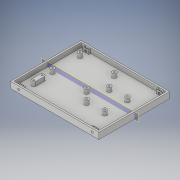
# Autodesk Inventor part: base
Saved by Autodesk Inventor 2017 (Build 210142000, 142)
## iProperties
Created: 2018-02-14
Part Number: base
Material: Generic
Document SubType Name: Modeling
Designer: chuck
Density: 1 g/cm^3
Appearance: Default
Author: chuck
Autodesk Inventor part; units mm, degrees
ref_plane "YZ Plane" through (0, 0, 0) normal (1, 0, 0) x (0, 1, 0)
ref_plane "XZ Plane" through (0, 0, 0) normal (0, 1, 0) x (-1, 0, 0)
ref_plane "XY Plane" through (0, 0, 0) normal (0, 0, 1) x (1, 0, 0)
sketch "Sketch1" plane through (0, 0, 0) normal (0, 1, 0) x (-1, 0, 0)
  line L0 (52.048, 52.048) -> (-82.4958, 52.048)
  line L1 (-82.4958, 52.048) -> (-82.4958, -55.394)
  line L2 (-82.4958, -55.394) -> (52.048, -55.394)
  line L3 (52.048, -55.394) -> (52.048, 52.048)
  line L4 (49.508, 49.508) -> (-79.9558, 49.508)
  line L5 (-79.9558, 49.508) -> (-79.9558, -52.854)
  line L6 (-79.9558, -52.854) -> (49.508, -52.854)
  line L7 (49.508, -52.854) -> (49.508, 49.508)
  point P0 (0, 0)
  dimension "d0" = 107.442
  dimension "d1" = 134.5438
  dimension "d2" = 2.54
  dimension "d3" = 2.54
  dimension "d4" = 2.54
  dimension "d5" = 2.54
  constraints: 16 end point, 4 parallel, 2 horizontal, 2 perpendicular
  measures "d0" distance of L2.end L0.start
  measures "d1" distance of L0.start L0.end
  measures "d2" distance between parallel lines of L2 L6
  measures "d3" distance between parallel lines of L3 L7
  measures "d4" distance between parallel lines of L0 L4
  measures "d5" distance between parallel lines of L1 L5
extrude "Extrusion1" add sketch "Sketch1" along normal blind 2.54 contours L3 L2 L1 L0 | L7 L6 L5 L4
sketch "Sketch4" plane through (0, 2.54, 0) normal (0, 1, 0) x (1, 0, 0)
  line L0 (82.4958, 55.394) -> (-52.048, 55.394)
  line L1 (-52.048, 55.394) -> (-52.048, -52.048)
  line L2 (-52.048, -52.048) -> (82.4958, -52.048)
  line L3 (82.4958, -52.048) -> (82.4958, 55.394)
  line L4 (79.9558, 52.854) -> (-49.508, 52.854)
  line L5 (-49.508, 52.854) -> (-49.508, -49.508)
  line L6 (-49.508, -49.508) -> (79.9558, -49.508)
  line L7 (79.9558, -49.508) -> (79.9558, 52.854)
  line L8 (82.4958, -52.048) -> (82.4958, 55.394) projected
  line L9 (82.4958, 55.394) -> (-52.048, 55.394) projected
  point P0 (0, 0)
  point P1 (0, 0)
  dimension "d8" = 107.442
  dimension "d9" = 134.5438
  dimension "d10" = 2.54
  dimension "d11" = 2.54
  dimension "d12" = 2.54
  dimension "d13" = 2.54
  dimension "d14" = 0
  dimension "d15" = 0
  constraints: 16 end point, 4 parallel, 2 horizontal, 2 perpendicular
  measures "d8" distance of L2.end L0.start
  measures "d9" distance of L0.start L0.end
  measures "d10" distance between parallel lines of L2 L6
  measures "d11" distance between parallel lines of L3 L7
  measures "d12" distance between parallel lines of L0 L4
  measures "d13" distance between parallel lines of L1 L5
  measures "d14" distance between parallel lines of L8 L3
  measures "d15" distance between parallel lines of L9 L0
extrude "Extrusion2" add sketch "Sketch4" along normal blind 6.985
sketch "Sketch5" plane through (-52.048, 0, 52.048) normal (0, 0, 1) x (1, 0, 0)
  circle A0 centre (12.7, 4.7625) radius 1.5875
  circle A1 centre (124.3838, 4.7625) radius 1.5875
  line L0 (0, 0) -> (134.5438, 0) projected
  line L1 (0, 0) -> (0, 9.525) projected
  line L2 (134.5438, 0) -> (134.5438, 9.525) projected
  point P0 (52.048, 0)
  dimension "d18" = 3.175
  dimension "d19" = 4.7625
  dimension "d20" = 4.7625
  dimension "d21" = 12.7
  dimension "d22" = 10.16
  constraints: 2 centre point, 1 equal radius
  measures "d18" diameter of A0
  measures "d19" distance from line of L0 A0.centre
  measures "d20" distance from line of L0 A1.centre
  measures "d21" distance from line of L1 A0.centre
  measures "d22" distance from line of L2 A1.centre
extrude "Extrusion3" cut sketch "Sketch5" against normal through all
sketch "Sketch6" plane through (0, 2.54, 0) normal (0, 1, 0) x (1, 0, 0)
  circle A0 centre (28.6445, 17.492) radius 3.175
  circle A1 centre (28.6445, -16.8742) radius 3.175
  circle A2 centre (56.3305, 17.492) radius 3.175
  circle A3 centre (56.3305, -16.8742) radius 3.175
  circle A4 centre (28.6445, 17.492) radius 1.143
  circle A5 centre (28.6445, -16.8742) radius 1.143
  circle A6 centre (56.3305, -16.8742) radius 1.143
  circle A7 centre (56.3305, 17.492) radius 1.143
  circle A8 centre (-37.9897, 39.7906) radius 3.175
  circle A9 centre (-37.9897, -2.1702) radius 3.175
  circle A10 centre (13.9787, 39.7906) radius 3.175
  circle A11 centre (13.9787, -2.1702) radius 3.175
  circle A12 centre (-37.9897, 39.7906) radius 1.143
  circle A13 centre (-37.9897, -2.1702) radius 1.143
  circle A14 centre (13.9787, -2.1702) radius 1.143
  circle A15 centre (13.9787, 39.7906) radius 1.143
  line L0 (-39.4169, -19.5919) -> (-39.4169, -32.2919)
  arc A16 (-39.4169, -32.2919) -> (-33.0669, -32.2919) centre (-36.2419, -32.2919) ccw
  arc A17 (-33.0669, -19.5919) -> (-39.4169, -19.5919) centre (-36.2419, -19.5919) ccw
  line L1 (-33.0669, -19.5919) -> (-33.0669, -32.2919)
  circle A18 centre (-36.2419, -19.5919) radius 1.143
  circle A19 centre (-36.2419, -32.2919) radius 1.143
  point P0 (0, 0)
  dimension "d25" = 0
  dimension "d26" = 0
  dimension "d27" = 0
  dimension "d28" = 0
  dimension "d29" = 0
  dimension "d30" = 0
  dimension "d31" = 0
  dimension "d32" = 0
  dimension "d67" = 51.9684
  dimension "d68" = 41.9608
  dimension "d69" = 34.3662
  dimension "d70" = 27.686
  dimension "d71" = 6.35
  dimension "d72" = 2.286
  dimension "d73" = 6.35
  dimension "d74" = 12.7
  constraints: 20 centre point, 16 equal radius, 10 coincident, 4 end point, 4 point on circle, 4 tangent, 2 vertical
  measures "d25" vertical distance of A2.centre A0.centre
  measures "d26" vertical distance of A3.centre A1.centre
  measures "d27" horizontal distance of A0.centre A1.centre
  measures "d28" horizontal distance of A2.centre A3.centre
  measures "d29" vertical distance of A10.centre A8.centre
  measures "d30" vertical distance of A11.centre A9.centre
  measures "d31" horizontal distance of A8.centre A9.centre
  measures "d32" horizontal distance of A10.centre A11.centre
  measures "d67" distance of A10.centre A8.centre
  measures "d68" distance of A8.centre A9.centre
  measures "d69" distance of A1.centre A0.centre
  measures "d70" distance of A2.centre A0.centre
  measures "d71" diameter of A8
  measures "d72" diameter of A12
  measures "d73" distance between parallel lines of L1 L0
  measures "d74" distance of A16.centre A17.centre
extrude "Extrusion4" add sketch "Sketch6" along normal blind 6.35
sketch "Sketch8" plane through (-49.508, 2.54, -52.854) normal (0, 0, 1) x (1, 0, 0)
  line L0 (6.985, 5.969) -> (6.985, 0.3894)
  line L1 (6.985, 0.3894) -> (10.16, -1.4437)
  line L2 (10.16, -1.4437) -> (13.335, 0.3894)
  line L3 (13.335, 0.3894) -> (13.335, 5.969)
  line L4 (13.335, 5.969) -> (14.859, 5.969)
  line L5 (14.859, 5.969) -> (14.859, -2.1406)
  line L6 (5.461, -2.1406) -> (5.461, 5.969)
  line L7 (5.461, 5.969) -> (6.985, 5.969)
  circle A0 centre (10.16, 2.2225) radius 1.5875
  line L8 (5.461, -2.1406) -> (14.859, -2.1406)
  line L9 (132.0038, 6.985) -> (-2.54, 6.985)
  circle A1 centre (121.8438, 2.2225) radius 1.5875
  line L10 (126.5428, 5.969) -> (126.5428, -2.1406)
  line L11 (125.0188, 5.969) -> (126.5428, 5.969)
  line L12 (125.0188, 0.3894) -> (125.0188, 5.969)
  line L13 (121.8438, -1.4437) -> (125.0188, 0.3894)
  line L14 (118.6688, 5.969) -> (118.6688, 0.3894)
  line L15 (117.1448, -2.1406) -> (126.5428, -2.1406)
  line L16 (117.1448, 5.969) -> (118.6688, 5.969)
  line L17 (117.1448, -2.1406) -> (117.1448, 5.969)
  line L18 (118.6688, 0.3894) -> (121.8438, -1.4437)
  line L19 (6.985, 5.969) -> (13.335, 5.969)
  line L20 (118.6688, 5.969) -> (125.0188, 5.969)
  point P0 (49.508, -2.54)
  point P1 (49.508, -2.54)
  dimension "d50" = 3.175
  dimension "d51" = 3.175
  dimension "d52" = 3.175
  dimension "d53" = 3.175
  dimension "d54" = 120
  dimension "d55" = 120
  dimension "d56" = 1.524
  dimension "d57" = 1.524
  dimension "d58" = 1.016
  dimension "d59" = 120
  dimension "d60" = 120
  dimension "d61" = 1.524
  dimension "d62" = 1.524
  constraints: 42 end point, 6 perpendicular, 4 parallel, 3 horizontal, 2 centre point, 2 point on line, 2 vertical, 1 coincident, 1 collinear
  measures "d50" distance from line of L0 A0.centre
  measures "d51" distance from line of L3 A0.centre
  measures "d52" distance from line of L1 A0.centre
  measures "d53" distance from line of A0.centre L2
  measures "d54" angle of L3 L2
  measures "d55" angle of L0 L1
  measures "d56" distance between parallel lines of L5 L3
  measures "d57" distance between parallel lines of L6 L0
  measures "d58" distance between parallel lines of L7 L9
  measures "d59" angle of L12 L13
  measures "d60" angle of L14 L18
  measures "d61" distance between parallel lines of L10 L12
  measures "d62" distance between parallel lines of L17 L14
extrude "Extrusion6" add sketch "Sketch8" along normal blind 3.048
sketch "Sketch7" plane through (-49.508, 2.54, -52.854) normal (0, 0, 1) x (1, 0, 0)
  line L0 (6.985, 5.969) -> (6.985, 0.3894)
  line L1 (6.985, 0.3894) -> (10.16, -1.4437)
  line L2 (10.16, -1.4437) -> (13.335, 0.3894)
  line L3 (13.335, 0.3894) -> (13.335, 5.969)
  line L4 (13.335, 5.969) -> (14.859, 5.969)
  line L5 (14.859, 5.969) -> (14.859, -2.1406)
  line L6 (5.461, -2.1406) -> (5.461, 5.969)
  line L7 (5.461, 5.969) -> (6.985, 5.969)
  circle A0 centre (10.16, 2.2225) radius 1.5875 projected
  line L8 (5.461, -2.1406) -> (14.859, -2.1406)
  line L9 (132.0038, 6.985) -> (-2.54, 6.985) projected
  circle A1 centre (121.8438, 2.2225) radius 1.5875 projected
  line L10 (118.6688, 5.969) -> (118.6688, 0.3894)
  line L11 (118.6688, 0.3894) -> (121.8438, -1.4437)
  line L12 (121.8438, -1.4437) -> (125.0188, 0.3894)
  line L13 (125.0188, 0.3894) -> (125.0188, 5.969)
  line L14 (125.0188, 5.969) -> (126.5428, 5.969)
  line L15 (126.5428, 5.969) -> (126.5428, -2.1406)
  line L16 (117.1448, -2.1406) -> (117.1448, 5.969)
  line L17 (117.1448, 5.969) -> (118.6688, 5.969)
  line L18 (117.1448, -2.1406) -> (126.5428, -2.1406)
  line L19 (6.985, 5.969) -> (13.335, 5.969)
  line L20 (118.6688, 5.969) -> (125.0188, 5.969)
  point P0 (49.508, -2.54)
  dimension "d35" = 3.175
  dimension "d36" = 3.175
  dimension "d37" = 3.175
  dimension "d38" = 3.175
  dimension "d39" = 120
  dimension "d40" = 120
  dimension "d41" = 1.524
  dimension "d42" = 1.524
  dimension "d43" = 1.016
  dimension "d44" = 120
  dimension "d45" = 120
  dimension "d46" = 1.524
  dimension "d47" = 1.524
  constraints: 40 end point, 6 perpendicular, 4 parallel, 3 horizontal, 2 point on line, 2 vertical, 1 coincident, 1 collinear
  measures "d35" distance from line of L0 A0.centre
  measures "d36" distance from line of L3 A0.centre
  measures "d37" distance from line of L1 A0.centre
  measures "d38" distance from line of A0.centre L2
  measures "d39" angle of L3 L2
  measures "d40" angle of L0 L1
  measures "d41" distance between parallel lines of L5 L3
  measures "d42" distance between parallel lines of L6 L0
  measures "d43" distance between parallel lines of L7 L9
  measures "d44" angle of L13 L12
  measures "d45" angle of L10 L11
  measures "d46" distance between parallel lines of L15 L13
  measures "d47" distance between parallel lines of L16 L10
extrude "Extrusion7" cut sketch "Sketch7" along normal blind 2.413 contours L19 L3 L2 L1 L0 | L20 L13 L12 L11 L10
ref_plane "Work Plane1" through (79.9558, 2.54, -1.673) normal (0, 0, -1) x (-1, 0, 0)
mirror "Mirror1" about plane through (79.9558, 2.54, -1.673) normal (0, 0, -1) of "Extrusion7", "Extrusion6"
body "Solid1"
